Autodesk Fusion 360 part; units mm, degrees
note: some values were not read from the file. Set by a fixed rule: which face or edge a step refers to.
(part 4 of 4)
  measures "d258" distance of P0 L5
  measures "d259" distance of P1 L7
extrude "Extrude3''" cut sketch "Sketch2 (4)" against normal blind 2.4 contours L0 L1 L2 L3 L4 L5 | L6 L7 L8 L9 L10 L11 | L12 L13 L14 L15 L16 L19 | L17 L18 L20 L21 L22 L23 | L24 L25 L26 L27 L28 L31 | L29 L30 L32 L33 L34 L35 | L36 L37 L38 L39 L40 L43 | L41 L42 L44 L45 L46 L47 | L48 L49 L50 L51 L52 L55 | L53 L54 L56 L57 L58 L59 | L60 L61 L62 L63 L64 L67 | L65 L66 L68 L69 L70 L71 | L72 L73 L74 L75 L76 L79 | L77 L78 L80 L81 L82 L83 | L84 L85 L86 L87 L88 L91 | L89 L90 L92 L93 L94 L95 | L96 L97 L98 L99 L100 L103 | L101 L102 L104 L105 L106 L107 | L108 L109 L110 L111 L112 L115 | L113 L114 L116 L117 L118 L119 | L120 L121 L122 L123 L124 L127 | L125 L126 L128 L129 L130 L131 | L132 L133 L134 L135 L136 L139 | L137 L138 L140 L141 L142 L143 | L144 L145 L146 L147 L148 L151 | L149 L150 L152 L153 L154 L155 | L156 L157 L158 L159 L160 L163 | L161 L162 L164 L165 L166 L167 | L168 L169 L170 L171 L172 L175 | L173 L174 L176 L177 L178 L179 | L180 L181 L182 L183 L184 L187 | L185 L186 L188 L189 L190 L191 | L192 L193 L194 L195 L196 L199 | L197 L198 L200 L201 L202 L203 | L204 L205 L206 L207 L208 L211 | L209 L210 L212 L213 L214 L215 | L216 L217 L218 L219 L220 L223 | L221 L222 L224 L225 L226 L227 | L228 L229 L230 L231 L232 L235 | L233 L234 L236 L237 L238 L239 | L240 L241 L242 L243 L244 L247 | L245 L246 L248 L249 L250 L251 | L252 L253 L254 L255 L256 L259 | L257 L258 L260 L261 L262 L263 | L264 L265 L266 L267 L268 L271 | L269 L270 L272 L273 L274 L275 | L276 L277 L278 L279 L280 L283 | L281 L282 L284 L285 L286 L287 | L288 L289 L290 L291 L292 L295 | L293 L294 L296 L297 L298 L299 | L300 L301 L302 L303 L304 L307 | L305 L306 L308 L309 L310 L311 | L312 L313 L314 L315 L316 L319 | L317 L318 L320 L321 L322 L323 | L324 L325 L326 L327 L328 L331 | L329 L330 L332 L333 L334 L335 | L336 L337 L338 L339 L340 L343 | L341 L342 L344 L345 L346 L347 | L348 L349 L350 L351 L352 L355 | L353 L354 L356 L357 L358 L359 | L360 L361 L362 L363 L364 L367 | L365 L366 L368 L369 L370 L371 | L372 L373 L374 L375 L376 L379 | L377 L378 L380 L381 L382 L383 | L384 L385 L386 L387 L388 L391 | L389 L390 L392 L393 L394 L395 | L396 L397 L398 L399 L400 L403 | L401 L402 L404 L405 L406 L407 | L408 L409 L410 L411 L412 L415 | L413 L414 L416 L417 L418 L419 | L420 L421 L422 L423 L424 L427 | L425 L426 L428 L429 L430 L431 | L432 L433 L434 L435 L436 L439 | L437 L438 L440 L441 L442 L443 | L444 L445 L446 L447 L448 L451 | L449 L450 L452 L453 L454 L455 | L456 L457 L458 L459 L460 L463 | L461 L462 L464 L465 L466 L467 | L468 L469 L470 L471 L472 L475 | L473 L474 L476 L477 L478 L479 | L480 L481 L482 L483 L484 L487 | L485 L486 L488 L489 L490 L491 | L492 L493 L494 L495 L496 L499 | L497 L498 L500 L501 L502 L503 | L504 L505 L506 L507 L508 L511 | L509 L510 L512 L513 L514 L515 | L516 L517 L518 L519 L520 L523 | L521 L522 L524 L525 L526 L527 | L528 L529 L530 L531 L532 L535 | L533 L534 L536 L537 L538 L539 | L540 L541 L542 L543 L544 L547 | L545 L546 L548 L549 L550 L551 | L552 L553 L554 L555 L556 L559 | L557 L558 L560 L561 L562 L563 | L564 L565 L566 L567 L568 L571 | L569 L570 L572 L573 L574 L575 | L576 L577 L578 L579 L580 L583 | L581 L582 L584 L585 L586 L587 | L588 L589 L590 L591 L592 L595 | L593 L594 L596 L597 L598 L599 | L600 L601 L602 L603 L604 L607 | L605 L606 L608 L609 L610 L611 | L612 L613 L614 L615 L616 L619 | L617 L618 L620 L621 L622 L623 | L624 L625 L626 L627 L628 L631 | L629 L630 L632 L633 L634 L635 | L636 L637 L638 L639 L640 L643 | L641 L642 L644 L645 L646 L647 | L648 L649 L650 L651 L652 L655 | L653 L654 L656 L657 L658 L659 | L660 L661 L662 L663 L664 L667 | L665 L666 L668 L669 L670 L671 | L672 L673 L674 L675 L676 L679 | L677 L678 L680 L681 L682 L683 | L684 L685 L686 L687 L688 L691 | L689 L690 L692 L693 L694 L695 | L696 L697 L698 L699 L700 L703 | L701 L702 L704 L705 L706 L707 | L708 L709 L710 L711 L712 L715 | L713 L714 L716 L717 L718 L719 | L720 L721 L722 L723 L724 L727 | L725 L726 L728 L729 L730 L731 | L732 L733 L734 L735 L736 L739 | L737 L738 L740 L741 L742 L743 | L744 L745 L746 L747 L748 L751 | L749 L750 L752 L753 L754 L755 | L756 L757 L758 L759 L760 L763 | L761 L762 L764 L765 L766 L767 | L768 L769 L770 L771 L772 L775 | L773 L774 L776 L777 L778 L779 | L780 L781 L782 L783 L784 L787 | L785 L786 L788 L789 L790 L791 | L792 L793 L794 L795 L796 L799 | L797 L798 L800 L801 L802 L803 | L804 L805 L806 L807 L808 L811 | L809 L810 L812 L813 L814 L815 | L816 L817 L818 L819 L820 L823 | L821 L822 L824 L825 L826 L827 | L828 L829 L830 L831 L832 L835 | L833 L834 L836 L837 L838 L839 bodies 4 in component "M5xxx-lid"
chamfer "Chamfer4" distance 0.8 angle 60 8 edges at (-106.2678, -69.2678, 54.4) (-1, -70, 54.4) (104.2678, -69.2678, 54.4) (105, 0, 54.4) (104.2678, 69.2678, 54.4) (-1, 70, 54.4) (-106.2678, 69.2678, 54.4) (-107, 0, 54.4) measured on face at (-106.8209, -68.4292, 57.0667) measured on face at (33.5, -74, 54.4) measured on face at (102.619, -69.9972, 57.0667) measured on face at (33.5, -74, 54.4) measured on face at (104.8209, 68.4292, 57.0667) measured on face at (33.5, -74, 54.4) measured on face at (-106.9972, 67.619, 57.0667) measured on face at (33.5, -74, 54.4) on bodies 4 in component "M5xxx-lid"
sketch "Sketch3 (3)" plane through (0, -76, 0) normal (0, -1, 0) x (1, 0, 0) in component "M5xxx-lid"
  line L0 (105, 58.4) -> (-107, 58.4)
  line L1 (-107, 58.4) -> (-107, 54.4)
  line L2 (-107, 54.4) -> (105, 54.4)
  line L3 (105, 54.4) -> (105, 58.4)
  line L4 (-26.6077, 39.2) -> (-10.4641, 39.2) construction
  line L5 (-18.5359, 39.2) -> (-18.5359, 58.4) construction
  line L6 (-17.7859, 47.101) -> (-17.0359, 48.4)
  line L7 (-17.0359, 48.4) -> (-17.7859, 49.699)
  line L8 (-17.7859, 49.699) -> (-19.2859, 49.699)
  line L9 (-19.2859, 49.699) -> (-20.0359, 48.4)
  line L10 (-20.0359, 48.4) -> (-19.2859, 47.101)
  line L11 (-19.2859, 47.101) -> (-17.7859, 47.101)
  line L12 (-107, 58.4) -> (106, 58.4)
  line L13 (-13.5359, 44.4) -> (-23.5359, 44.4)
  line L14 (-23.5359, 44.4) -> (-23.5359, 54.4)
  line L15 (-23.5359, 54.4) -> (-13.5359, 54.4)
  line L16 (-13.5359, 54.4) -> (-13.5359, 44.4)
  line L17 (-13.5359, 44.4) -> (-23.5359, 54.4) construction
  line L18 (-23.5359, 44.4) -> (-13.5359, 54.4) construction
  point P0 (-26.6077, 39.2)
  point P1 (-10.4641, 39.2)
  point P2 (-18.5359, 48.4)
  point P3 (-18.5359, 49.4)
  dimension "d280" = 1.5
  dimension "d281" = 10
  dimension "d282" = 10
  dimension "d283" = 10
  constraint coincident P0 L4.start
  constraint coincident P1 L4.end
  constraint midpoint L4 L5.start
  constraint coincident L0 L5.end
  constraint perpendicular L0 L5
  constraint horizontal L11
  constraint coincident L5 P2
  constraint perpendicular L13 L14
  constraint parallel L13 L15
  constraint parallel L14 L16
  constraint horizontal L13
  constraint coincident L17 P3
  constraint coincident L18 P3
  constraint coincident L5 P3
  constraint coincident L2 L15.end
  measures "d280" distance of L6.start P2
  measures "d281" distance of P2 L12
  measures "d282" distance of L13.start L13.end
  measures "d283" distance of L13.start L15.end
extrude "Extrude6'''" add sketch "Sketch3 (3)" against normal blind 4 contours L2 L13 L14 L15 L16 bodies 4 in component "M5xxx-lid"
extrude "Extrude7''" add 1 faces at (-18.2859, -72, 52.833) along direction (0, -1, 0) blind 4 from surface at -148 on bodies 4 bodies 4 in component "M5xxx-lid"
fillet "Fillet2'" radius 2.5 8 edges at (-13.5359, -74, 54.4) (-13.5359, -74, 44.4) (-23.5359, -74, 44.4) (-23.5359, -74, 54.4) (-23.5359, 74, 44.4) (-23.5359, 74, 54.4) (-13.5359, 74, 44.4) (-13.5359, 74, 54.4) on bodies 4 in component "M5xxx-lid"
chamfer "Chamfer5'" distance 0.8 angle 45 24 edges at (111, 0, 54.4) (109.2426, -74.2426, 54.4) (46.9821, -76, 54.4) (-12.8037, -76, 53.6678) (-13.5359, -76, 49.4) (-14.2681, -76, 45.1322) (-18.5359, -76, 44.4) (-22.8037, -76, 45.1322) (-23.5359, -76, 49.4) (-24.2681, -76, 53.6678) (-66.5179, -76, 54.4) (-111.2426, -74.2426, 54.4) (-113, 0, 54.4) (-111.2426, 74.2426, 54.4) (-66.5179, 76, 54.4) (-24.2681, 76, 53.6678) (-23.5359, 76, 49.4) (-22.8037, 76, 45.1322) (-18.5359, 76, 44.4) (-14.2681, 76, 45.1322) (-13.5359, 76, 49.4) (-12.8037, 76, 53.6678) (46.9821, 76, 54.4) (109.2426, 74.2426, 54.4) on bodies 4 in component "M5xxx-lid"
sketch "Sketch17" plane through (0, 78.4, 0) normal (0, 1, 0) x (-1, 0, 0) in component "M5xxx-base"
  line L0 (30.0718, 0) -> (26.6077, 6)
  line L1 (26.6077, 6) -> (30.0718, 12)
  line L2 (30.0718, 12) -> (37, 12)
  line L3 (37, 12) -> (40.4641, 6)
  line L4 (40.4641, 6) -> (37, 0)
  line L5 (37, 0) -> (30.0718, 0)
  line L6 (90.0718, 33.2) -> (86.6077, 39.2)
  line L7 (86.6077, 39.2) -> (90.0718, 45.2)
  line L8 (90.0718, 45.2) -> (97, 45.2)
  line L9 (97, 45.2) -> (100.4641, 39.2)
  line L10 (100.4641, 39.2) -> (97, 33.2)
  line L11 (97, 33.2) -> (90.0718, 33.2)
  line L12 (0.0718, 16.6) -> (-3.3923, 22.6)
  line L13 (-3.3923, 22.6) -> (0.0718, 28.6)
  line L14 (0.0718, 28.6) -> (7, 28.6)
  line L15 (7, 28.6) -> (10.4641, 22.6)
  line L16 (10.4641, 22.6) -> (7, 16.6)
  line L17 (7, 16.6) -> (0.0718, 16.6)
  line L18 (0.0718, 33.2) -> (-3.3923, 39.2)
  line L19 (-3.3923, 39.2) -> (0.0718, 45.2)
  line L20 (0.0718, 45.2) -> (7, 45.2)
  line L21 (7, 45.2) -> (10.4641, 39.2)
  line L22 (10.4641, 39.2) -> (7, 33.2)
  line L23 (7, 33.2) -> (0.0718, 33.2)
  line L24 (90.0718, 16.6) -> (86.6077, 22.6)
  line L25 (86.6077, 22.6) -> (90.0718, 28.6)
  line L26 (90.0718, 28.6) -> (97, 28.6)
  line L27 (97, 28.6) -> (100.4641, 22.6)
  line L28 (100.4641, 22.6) -> (97, 16.6)
  line L29 (97, 16.6) -> (90.0718, 16.6)
  line L30 (30.0718, 16.6) -> (26.6077, 22.6)
  line L31 (26.6077, 22.6) -> (30.0718, 28.6)
  line L32 (30.0718, 28.6) -> (37, 28.6)
  line L33 (37, 28.6) -> (40.4641, 22.6)
  line L34 (40.4641, 22.6) -> (37, 16.6)
  line L35 (37, 16.6) -> (30.0718, 16.6)
  line L36 (60.0718, 0) -> (56.6077, 6)
  line L37 (56.6077, 6) -> (60.0718, 12)
  line L38 (60.0718, 12) -> (67, 12)
  line L39 (67, 12) -> (70.4641, 6)
  line L40 (70.4641, 6) -> (67, 0)
  line L41 (67, 0) -> (60.0718, 0)
  line L42 (60.0718, 33.2) -> (56.6077, 39.2)
  line L43 (56.6077, 39.2) -> (60.0718, 45.2)
  line L44 (60.0718, 45.2) -> (67, 45.2)
  line L45 (67, 45.2) -> (70.4641, 39.2)
  line L46 (70.4641, 39.2) -> (67, 33.2)
  line L47 (67, 33.2) -> (60.0718, 33.2)
  line L48 (0.0718, 0) -> (-3.3923, 6)
  line L49 (-3.3923, 6) -> (0.0718, 12)
  line L50 (0.0718, 12) -> (7, 12)
  line L51 (7, 12) -> (10.4641, 6)
  line L52 (10.4641, 6) -> (7, 0)
  line L53 (7, 0) -> (0.0718, 0)
  line L54 (30.0718, 33.2) -> (26.6077, 39.2)
  line L55 (26.6077, 39.2) -> (30.0718, 45.2)
  line L56 (30.0718, 45.2) -> (37, 45.2)
  line L57 (37, 45.2) -> (40.4641, 39.2)
  line L58 (40.4641, 39.2) -> (37, 33.2)
  line L59 (37, 33.2) -> (30.0718, 33.2)
  line L60 (60.0718, 16.6) -> (56.6077, 22.6)
  line L61 (56.6077, 22.6) -> (60.0718, 28.6)
  line L62 (60.0718, 28.6) -> (67, 28.6)
  line L63 (67, 28.6) -> (70.4641, 22.6)
  line L64 (70.4641, 22.6) -> (67, 16.6)
  line L65 (67, 16.6) -> (60.0718, 16.6)
  line L66 (86.6077, 6) -> (90.0718, 12)
  line L67 (90.0718, 12) -> (97, 12)
  line L68 (97, 12) -> (100.4641, 6)
  line L69 (100.4641, 6) -> (97, 0)
  line L70 (97, 0) -> (90.0718, 0)
  line L71 (90.0718, 0) -> (86.6077, 6)
  line L72 (-106, -6.1359) -> (107, -6.1359)
  line L73 (107, -6.1359) -> (107, 58.4)
  line L74 (107, 58.4) -> (-106, 58.4)
  line L75 (-106, 58.4) -> (-106, -6.1359)
  circle A0 centre (18.5359, 48.4) radius 1.6
  point P0 (18.5359, 48.4)
  dimension "d291" = 3.2
  constraint coincident P0 A0.centre
  measures "d291" diameter of A0
extrude "Extrude24" cut sketch "Sketch17" against normal blind 156.8 contours A0 bodies 3 in component "M5xxx-base"
chamfer "Chamfer18" distance 2 angle 45 2 edges at (-17.0442, -78.4, 47.8214) (-17.0442, 78.4, 48.9786) on bodies 3 in component "M5xxx-base"
chamfer "Chamfer19" distance 1 angle 45 5 edges at (10.3384, -71.8081, -1.6) (-109.6616, -71.8081, -1.6) (100.3384, -71.8081, -1.6) (100.3384, 68.1919, -1.6) (-109.6616, 68.1919, -1.6) on bodies 3 in component "M5xxx-base"
extrude "Extrude8'" [suppressed] in component "PCB-M5000"
component "PCB-M5000" placed x (1, 0, 0) y (0, 1, 0) z (0, 0, 1) at (0, 0, 0)
component "PCB-M5000" placed x (1, 0, 0) y (0, 1, 0) z (0, 0, 1) at (0, 0, 16.6)
component "M2000" placed x (1, 0, 0) y (0, 1, 0) z (0, 0, 1) at (0, 0, 0)
component "M5xxx-base" placed x (1, 0, 0) y (0, 1, 0) z (0, 0, 1) at (0, 0, 0)
component "M5xxx-lid" placed x (1, 0, 0) y (0, 1, 0) z (0, 0, 1) at (0, 0, 0)
equation "d73 = 11 mm + ( ( 3.2 / 2 ) * 1 mm )"
equation "d87 = d86"
equation "d88 = d86"
equation "d89 = d86"
equation "d90 = d86"
named bodies: "m5000-pcb", "PCB-M2000", "M5000-base", "M5000-lid"
